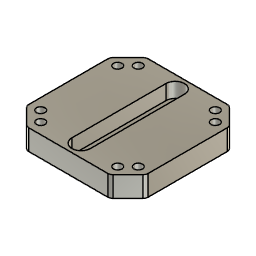
GPS_AMPS_PLATE (Autodesk Fusion 360 design; units mm, degrees)
Autodesk Fusion 360 part; units mm, degrees
sketch "Esquisse1" plane through (0, 0, 0) normal (0, 0, 1) x (1, 0, 0)
  line L0 (7.8284, 0) -> (38.6716, 0)
  line L1 (46.5, 7.8284) -> (46.5, 38.6716)
  line L2 (38.6716, 46.5) -> (7.8284, 46.5)
  line L3 (0, 38.6716) -> (0, 7.8284)
  circle A0 centre (8.25, 4.25) radius 1.65
  circle A1 centre (38.25, 4.25) radius 1.65
  circle A2 centre (8.25, 42.25) radius 1.65
  circle A3 centre (38.25, 42.25) radius 1.65
  circle A4 centre (4.25, 8.25) radius 1.65
  circle A5 centre (42.25, 8.25) radius 1.65
  circle A6 centre (4.25, 38.25) radius 1.65
  circle A7 centre (42.25, 38.25) radius 1.65
  line L4 (40.0858, 0.5858) -> (45.9142, 6.4142)
  line L5 (6.4142, 0.5858) -> (0.5858, 6.4142)
  line L6 (45.9142, 40.0858) -> (40.0858, 45.9142)
  line L7 (6.4142, 45.9142) -> (0.5858, 40.0858)
  arc A8 (46.5, 38.6716) -> (45.9142, 40.0858) centre (44.5, 38.6716) ccw
  arc A9 (40.0858, 45.9142) -> (38.6716, 46.5) centre (38.6716, 44.5) ccw
  arc A10 (7.8284, 46.5) -> (6.4142, 45.9142) centre (7.8284, 44.5) ccw
  arc A11 (0.5858, 40.0858) -> (0, 38.6716) centre (2, 38.6716) ccw
  arc A12 (0, 7.8284) -> (0.5858, 6.4142) centre (2, 7.8284) ccw
  arc A13 (6.4142, 0.5858) -> (7.8284, 0) centre (7.8284, 2) ccw
  arc A14 (38.6716, 0) -> (40.0858, 0.5858) centre (38.6716, 2) ccw
  arc A15 (45.9142, 6.4142) -> (46.5, 7.8284) centre (44.5, 7.8284) ccw
  line L8 (19.5, 41.5) -> (19.5, 5)
  arc A16 (19.5, 5) -> (27, 5) centre (23.25, 5) ccw
  line L9 (27, 5) -> (27, 41.5)
  arc A17 (27, 41.5) -> (19.5, 41.5) centre (23.25, 41.5) ccw
  line L10 (23.25, 45.25) -> (23.25, 1.25) construction
  line L11 (21.25, 41.5) -> (21.25, 5)
  arc A18 (21.25, 5) -> (25.25, 5) centre (23.25, 5) ccw
  line L12 (25.25, 5) -> (25.25, 41.5)
  arc A19 (25.25, 41.5) -> (21.25, 41.5) centre (23.25, 41.5) ccw
  line L13 (23.25, 41.5) -> (23.25, 5) construction
  point P0 (46.5, 0)
  point P1 (46.5, 46.5)
  point P2 (0, 46.5)
  point P3 (39.5, 0)
  point P4 (46.5, 7)
  point P5 (7, 0)
  point P6 (0, 7)
  point P7 (46.5, 39.5)
  point P8 (39.5, 46.5)
  point P9 (7, 46.5)
  point P10 (0, 39.5)
  dimension "d1" = 46.5
  dimension "d2" = 46.5
  dimension "d3" = 3.3
  dimension "d4" = 4.25
  dimension "d5" = 8.25
  dimension "d8" = 30
  dimension "d9" = 38
  dimension "d10" = 3.3
  dimension "d11" = 8.25
  dimension "d12" = 4.25
  dimension "d15" = 38
  dimension "d16" = 30
  dimension "d17" = 7
  dimension "d18" = 7
  dimension "d19" = 7
  dimension "d20" = 7
  dimension "d21" = 7
  dimension "d22" = 7
  dimension "d23" = 7
  dimension "d24" = 7
  dimension "d25" = 2
  dimension "d26" = 7.5
  dimension "d27" = 44
  dimension "d28" = 23.25
  dimension "d29" = 1.25
  dimension "d30" = 4
  constraint horizontal L0
  constraint vertical L1
  constraint horizontal L2
  constraint vertical L3
  constraint coincident P0 L0
  constraint coincident P0 L1
  constraint coincident origin L0
  constraint coincident origin L3
  constraint coincident P1 L1
  constraint coincident P1 L2
  constraint coincident P2 L2
  constraint coincident P2 L3
  constraint coincident P7 L6
  constraint coincident L1 P7
  constraint tangent L6 A8
  constraint tangent L1 A8
  constraint coincident P8 L6
  constraint coincident L2 P8
  constraint tangent L6 A9
  constraint tangent L2 A9
  constraint equal A8 A9
  constraint coincident P9 L7
  constraint coincident L2 P9
  constraint tangent L7 A10
  constraint tangent L2 A10
  constraint equal A8 A10
  constraint coincident P10 L7
  constraint coincident L3 P10
  constraint tangent L7 A11
  constraint tangent L3 A11
  constraint equal A8 A11
  constraint coincident P6 L5
  constraint coincident L3 P6
  constraint tangent L5 A12
  constraint tangent L3 A12
  constraint equal A8 A12
  constraint coincident P5 L5
  constraint coincident L0 P5
  constraint tangent L5 A13
  constraint tangent L0 A13
  constraint equal A8 A13
  constraint coincident P3 L4
  constraint coincident L0 P3
  constraint tangent L4 A14
  constraint tangent L0 A14
  constraint equal A8 A14
  constraint coincident P4 L4
  constraint coincident L1 P4
  constraint tangent L4 A15
  constraint tangent L1 A15
  constraint equal A8 A15
  constraint tangent L8 A16
  constraint tangent A16 L9
  constraint parallel L8 L9
  constraint tangent L9 A17
  constraint tangent L8 A17
  constraint midpoint A17 L10.start
  constraint midpoint A16 L10.end
  constraint vertical L10
  constraint tangent L11 A18
  constraint tangent A18 L12
  constraint parallel L11 L12
  constraint tangent L12 A19
  constraint tangent L11 A19
  constraint coincident A16.centre A18.centre
  constraint parallel L10 L13
  constraint coincident A17.centre A19.centre
  measures "d1" distance of origin P0
  measures "d2" distance of origin P2
  measures "d3" diameter of A0
  measures "d4" distance of L0 A0.centre
  measures "d5" distance of L3 A0.centre
  measures "d10" diameter of A4
  measures "d11" distance of L0 A4.centre
  measures "d12" distance of L3 A4.centre
  measures "d17" distance of P0 P3
  measures "d18" distance of P0 P4
  measures "d19" distance of origin P5
  measures "d20" distance of origin P6
  measures "d21" distance of P1 P7
  measures "d22" distance of P1 P8
  measures "d23" distance of P2 P9
  measures "d24" distance of P2 P10
  measures "d25" radius of A8
  measures "d26" diameter of A16
  measures "d27" distance of L10.start L10.end
  measures "d28" distance of L1 L10
  measures "d29" distance of L2 L10.start
  measures "d30" diameter of A18
extrude "Extrusion1" add sketch "Esquisse1" along normal blind 8 contours L0 L1 L2 L3 L4 L5 L6 L7 A8 A9 A10 A11 A12 A13 A14 A15 | L8 A16 L9 A17
sketch "Esquisse2" plane through (0, 0, 8) normal (0, 0, 1) x (-1, 0, 0)
  circle A0 centre (-38.25, -4.25) radius 1.65
  circle A1 centre (-38.25, -42.25) radius 1.65
  arc A2 (-25.25, -41.5) -> (-21.25, -41.5) centre (-23.25, -41.5) ccw
  line L0 (-25.25, -41.5) -> (-25.25, -5)
  arc A3 (-21.25, -5) -> (-25.25, -5) centre (-23.25, -5) ccw
  line L1 (-21.25, -5) -> (-21.25, -41.5)
  circle A4 centre (-4.25, -38.25) radius 1.65
  circle A5 centre (-42.25, -38.25) radius 1.65
  circle A6 centre (-4.25, -8.25) radius 1.65
  circle A7 centre (-42.25, -8.25) radius 1.65
  circle A8 centre (-8.25, -42.25) radius 1.65
  circle A9 centre (-8.25, -4.25) radius 1.65
  arc A10 (-6.4142, -0.5858) -> (-7.8284, 0) centre (-7.8284, -2) ccw
  line L2 (-7.8284, 0) -> (-38.6716, 0)
  arc A11 (-38.6716, 0) -> (-40.0858, -0.5858) centre (-38.6716, -2) ccw
  line L3 (-40.0858, -0.5858) -> (-45.9142, -6.4142)
  arc A12 (-45.9142, -6.4142) -> (-46.5, -7.8284) centre (-44.5, -7.8284) ccw
  line L4 (-46.5, -7.8284) -> (-46.5, -38.6716)
  arc A13 (-46.5, -38.6716) -> (-45.9142, -40.0858) centre (-44.5, -38.6716) ccw
  line L5 (-45.9142, -40.0858) -> (-40.0858, -45.9142)
  arc A14 (-40.0858, -45.9142) -> (-38.6716, -46.5) centre (-38.6716, -44.5) ccw
  line L6 (-38.6716, -46.5) -> (-7.8284, -46.5)
  arc A15 (-7.8284, -46.5) -> (-6.4142, -45.9142) centre (-7.8284, -44.5) ccw
  line L7 (-6.4142, -45.9142) -> (-0.5858, -40.0858)
  arc A16 (-0.5858, -40.0858) -> (0, -38.6716) centre (-2, -38.6716) ccw
  line L8 (0, -38.6716) -> (0, -7.8284)
  arc A17 (0, -7.8284) -> (-0.5858, -6.4142) centre (-2, -7.8284) ccw
  line L9 (-0.5858, -6.4142) -> (-6.4142, -0.5858)
  line L10 (-19.65, -41.65) -> (-19.65, -5)
  arc A18 (-19.65, -5) -> (-26.85, -5) centre (-23.25, -5) ccw
  line L11 (-26.85, -5) -> (-26.85, -41.65)
  arc A19 (-26.85, -41.65) -> (-19.65, -41.65) centre (-23.25, -41.65) ccw
  line L12 (-23.25, -45.25) -> (-23.25, -1.4) construction
  dimension "d33" = 7.2
  dimension "d34" = 1.25
  dimension "d35" = 23.25
  constraint tangent L10 A18
  constraint tangent A18 L11
  constraint parallel L10 L11
  constraint tangent L11 A19
  constraint tangent L10 A19
  constraint midpoint A19 L12.start
  constraint midpoint A18 L12.end
  constraint parallel L0 L12
  measures "d33" diameter of A18
  measures "d34" distance of L6 L12.start
  measures "d35" distance of L8 L12
extrude "Extrusion2" cut sketch "Esquisse2" against normal blind 5.75 contours L10 A18 L11 A19
equation "d18 = d17"
equation "d20 = d19"
equation "d22 = d21"
equation "d24 = d23"
equation "d28 = ( 46.5 / 2 ) * 1 mm"
equation "d29 = ( 2.5 / 2 ) * 1 mm"
